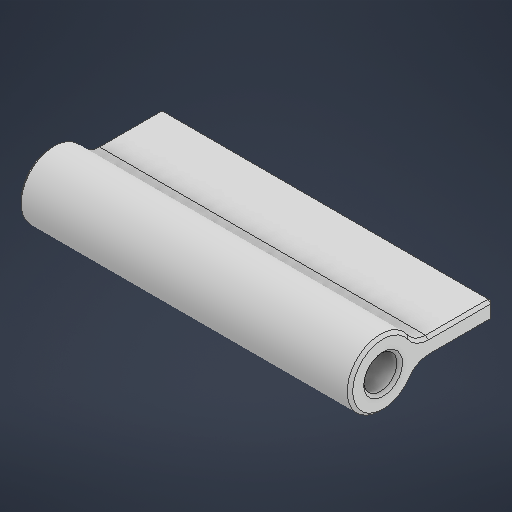
# Autodesk Inventor part: CoinLockUpperRow
Saved by Autodesk Inventor 2026.3 (Build 303398000, 398)
## iProperties
Created: 2026-05-05
Part Number: CoinLockUpperRow
Material: Generic
Document SubType Name: Modeling
Designer: frede
Density: 1 g/cm^3
Appearance: Default
Author: frede
Autodesk Inventor part; units mm, degrees
ref_plane "YZ Plane" through (0, 0, 0) normal (1, 0, 0) x (0, 1, 0)
ref_plane "XZ Plane" through (0, 0, 0) normal (0, 1, 0) x (-1, 0, 0)
ref_plane "XY Plane" through (0, 0, 0) normal (0, 0, 1) x (1, 0, 0)
sketch "Sketch3" plane through (0, 0, 0) normal (1, 0, 0) x (0, 1, 0)
  circle A0 centre (0, 0) radius 1.5
  arc A1 (1.725, -2.4545) -> (-1.6531, -2.5034) centre (0, 0) ccw
  line L0 (-0.7552, -4.1724) -> (-0.7552, -10)
  line L1 (-0.7552, -10) -> (0.875, -10)
  line L2 (0.875, -10) -> (0.875, -4.0908)
  arc A2 (1.725, -2.4545) -> (0.875, -4.0908) centre (2.875, -4.0908) ccw
  arc A3 (-0.7552, -4.1724) -> (-1.6531, -2.5034) centre (-2.7552, -4.1724) ccw
  dimension "d4" = 3
  dimension "d5" = 6
  dimension "d7" = 2
  constraints: 6 end point, 6 point on circle, 4 centre point, 4 tangent, 2 coincident, 1 equal radius, 1 parallel
  measures "d4" diameter of A0
  measures "d5" diameter of A1
  measures "d7" radius of A2
extrude "Extrusion2" add sketch "Sketch3" along normal blind 30
chamfer "Chamfer1" distance 0.25 angle 45 16 edges at (30, 0.875, -7.0454) (30, 1.1002, -3.1688) (30, -0.0435, 2.9997) (30, -0.9939, -3.2248) (30, -0.7552, -7.0862) (30, 0.0599, -10) (30, -1.5, 0) (0, -1.5, 0) (0, -0.0435, 2.9997) (0, -0.9939, -3.2248) (0, -0.7552, -7.0862) (0, 1.1002, -3.1688) (0, 0.875, -7.0454) (0, 0.0599, -10) (15, 0.875, -10) (15, -0.7552, -10)
body "Solid2"
